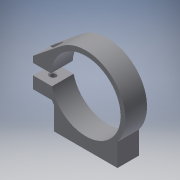
# Autodesk Inventor part: MotorClampXT
Saved by Autodesk Inventor 2017 (Build 210142000, 142)
## iProperties
Created: 2015-08-05
Part Number: MotorClampXT
Material: Generic
Document SubType Name: Modeling
Designer: Dale
Density: 1 g/cm^3
Appearance: Default
Author: Dale
Autodesk Inventor part; units mm, degrees
ref_plane "YZ Plane" through (0, 0, 0) normal (1, 0, 0) x (0, 1, 0)
ref_plane "XZ Plane" through (0, 0, 0) normal (0, 1, 0) x (-1, 0, 0)
ref_plane "XY Plane" through (0, 0, 0) normal (0, 0, 1) x (1, 0, 0)
sketch "Sketch1" plane through (0, 0, 0) normal (0, 0, 1) x (1, 0, 0)
  arc A0 (-1.1319, 20.1168) -> (-1.6326, 25.8318) centre (16.7386, 24.5618) ccw
  line L0 (0, 0) -> (33.4772, 0)
  line L1 (33.4772, 0) -> (33.4772, 11.955)
  line L2 (0, 0) -> (0, 11.955)
  line L3 (-1.2219, 13.7668) -> (-11.2014, 13.7668)
  line L4 (-11.2014, 13.7668) -> (-11.2014, 20.1168)
  line L5 (-11.2014, 20.1168) -> (-1.1319, 20.1168)
  line L6 (-11.2014, 25.8318) -> (-1.6326, 25.8318)
  line L7 (-11.2014, 25.8318) -> (-11.2014, 29.0068)
  line L8 (-11.2014, 29.0068) -> (3.6223, 40.9042)
  arc A1 (-1.2219, 13.7668) -> (0, 11.955) centre (16.7386, 24.5618) ccw
  arc A2 (33.4772, 11.955) -> (3.6223, 40.9042) centre (16.7386, 24.5618) ccw
  dimension "d0" = 24.5618
  dimension "d1" = 16.7386
  dimension "d2" = 36.83
  dimension "d4" = 33.4772
  dimension "d5" = 11.955
  dimension "d6" = 6.35
  dimension "d7" = 13.7668
  dimension "d8" = 5.715
  dimension "d9" = 27.94
  dimension "d10" = 3.175
  dimension "d13" = 20.955
  constraints: 18 end point, 6 point on circle, 4 horizontal, 4 vertical, 3 centre point, 1 coincident, 1 collinear, 1 parallel, 1 tangent
  measures "d0" vertical distance of L0.start A1.centre
  measures "d1" horizontal distance of A0.centre L0.start
  measures "d2" diameter of A0
  measures "d4" distance of L0.start L0.end
  measures "d5" distance of L0.end L1.end
  measures "d6" distance of L3.end L4.end
  measures "d7" distance from line of L0.start L3
  measures "d8" distance between parallel lines of L5 L6
  measures "d9" distance from line of L4 A0.centre
  measures "d10" distance of L6.start L7.end
  measures "d13" radius of A2
extrude "Clamp Body" add sketch "Sketch1" along normal blind 11.43
sketch "Sketch2" plane through (0, 0, 0) normal (0, -1, 0) x (1, 0, 0)
  circle A0 centre (3.2512, 5.715) radius 1.5
  circle A1 centre (30.2006, 5.715) radius 1.5
  line L0 (-11.2014, 0) -> (-1.2219, 0) projected
  line L1 (0, 0) -> (0, 11.43) projected
  line L2 (33.4772, 0) -> (33.4772, 11.43) projected
  dimension "d16" = 3
  dimension "d17" = 5.715
  dimension "d18" = 26.9494
  dimension "d20" = 3.2512
  dimension "d21" = 3.2766
  constraints: 2 centre point, 1 equal radius, 1 horizontal alignment
  measures "d16" diameter of A0
  measures "d17" distance from line of A0.centre L0
  measures "d18" distance of A1.centre A0.centre
  measures "d20" distance from line of A0.centre L1
  measures "d21" distance from line of L2 A1.centre
hole "Mounting Holes" at (30.2006, 0, 5.715) at (3.2512, 0, 5.715) direction (0, 1, 0) diameter 3 depth 9.525 tip angle 118 countersink diameter 4 countersink angle 90
sketch "Sketch7" plane through (-11.2014, 20.1168, 0) normal (0, 1, 0) x (1, 0, 0)
  circle A0 centre (5.08, -5.715) radius 1.5
  line L0 (0, 0) -> (0, -11.43) projected
  line L1 (10.0695, 0) -> (0, 0) projected
  point P0 (11.2014, 0)
  dimension "d41" = 3
  dimension "d42" = 5.08
  dimension "d43" = 5.715
  constraints: 1 centre point
  measures "d41" diameter of A0
  measures "d42" distance from line of A0.centre L0
  measures "d43" distance from line of L1 A0.centre
hole "Tightner Threaded Hole" at (-6.1214, 20.1168, 5.715) direction (0, -1, 0) diameter 3 end through all countersink diameter 4 countersink angle 90
sketch "Sketch4" plane through (-11.2014, 25.8318, 0) normal (0, -1, 0) x (1, 0, 0)
  circle A0 centre (5.08, 5.715) radius 1.95
  circle A1 centre (5.08, 5.715) radius 1.5 projected
  point P0 (11.2014, 0)
  dimension "d31" = 3.9
  constraints: 1 centre point, 1 concentric
  measures "d31" diameter of A0
extrude "Tightner Hole" cut sketch "Sketch4" against normal blind 9.525 contours A0 | A1
sketch "Sketch6" plane through (-11.2014, 25.8318, 0) normal (-1, 0, 0) x (0, 0, 1)
  line L0 (2.413, 3.175) -> (9.017, 3.175)
  line L1 (9.017, 3.175) -> (9.017, 15.875)
  line L2 (9.017, 15.875) -> (2.413, 15.875)
  line L3 (2.413, 15.875) -> (2.413, 3.175)
  line L4 (0, 3.175) -> (0, 0) projected
  line L5 (11.43, 3.175) -> (11.43, 0) projected
  line L6 (0, 3.175) -> (11.43, 3.175) projected
  point P0 (0, -25.8318)
  dimension "d34" = 2.413
  dimension "d35" = 2.413
  dimension "d36" = 12.7
  dimension "d39" = 6.604
  constraints: 8 end point, 2 parallel, 1 collinear, 1 horizontal, 1 perpendicular
  measures "d34" distance between parallel lines of L3 L4
  measures "d35" distance between parallel lines of L1 L5
  measures "d36" distance between parallel lines of L2 L0
  measures "d39" distance between parallel lines of L3 L1
extrude "Tightner Cutout" cut sketch "Sketch6" against normal blind 8.89
fillet "Tightner Fillet" radius 3.175 2 edges at (-2.3114, 32.5743, 2.413) (-2.3114, 32.5743, 9.017)
body "Solid1"
